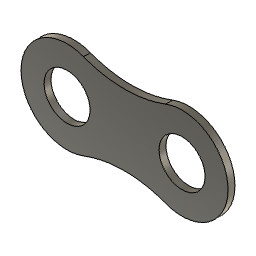
Chain Link (Autodesk Fusion 360 design; units mm, degrees)
Autodesk Fusion 360 part; units mm, degrees
sketch "Sketch1" plane through (0, 0, 0) normal (0, 1, 0) x (1, 0, 0)
  line L0 (0, 0) -> (50, 0) construction
  circle A0 centre (50, 0) radius 10
  circle A1 centre (0, 0) radius 10
  arc A2 (42.8571, -18.681) -> (7.1429, -18.681) centre (25, -65.3835) ccw
  arc A3 (7.1429, 18.681) -> (42.8571, 18.681) centre (25, 65.3835) ccw
  arc A4 (7.1429, 18.681) -> (7.1429, -18.681) centre (0, 0) ccw
  arc A5 (42.8571, -18.681) -> (42.8571, 18.681) centre (50, 0) ccw
  dimension "d13" = 50
  dimension "d14" = 40
  dimension "d15" = 40
  dimension "d16" = 20
  dimension "d17" = 20
  dimension "d18" = 100
  dimension "d19" = 100
  constraint coincident L0.start A1.centre
  constraint horizontal L0
  constraint coincident L0.end A0.centre
  constraint concentric A0 A5
  constraint tangent A2 A4
  constraint tangent A2 A5
  constraint tangent A3 A4
  constraint tangent A3 A5
  measures "d13" distance of L0.start L0.end
  measures "d14" diameter of A4
  measures "d15" diameter of A5
  measures "d16" diameter of A0
  measures "d17" diameter of A1
  measures "d18" diameter of A2
  measures "d19" diameter of A3
extrude "Extrude1" add sketch "Sketch1" along normal blind 3
